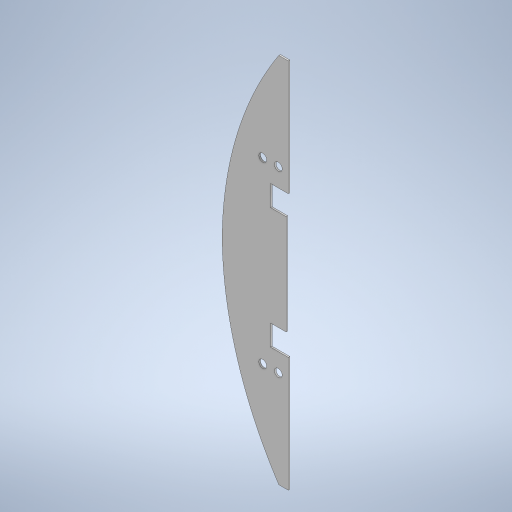
# Autodesk Inventor part: sensor2
Saved by Autodesk Inventor 2023 (Build 270158000, 158)
## iProperties
Created: 2023-08-10
Part Number: sensor2
Material: Genérico
Document SubType Name: Modeling
Designer: azeve
Density: 1 g/cm^3
Appearance: Padrão
Author: azeve
Autodesk Inventor part; units mm, degrees
ref_plane "YZ Plane" through (0, 0, 0) normal (1, 0, 0) x (0, 1, 0)
ref_plane "XZ Plane" through (0, 0, 0) normal (0, 1, 0) x (-1, 0, 0)
ref_plane "XY Plane" through (0, 0, 0) normal (0, 0, 1) x (1, 0, 0)
sketch "Esboço1" plane through (0, 0, 0) normal (0, 0, 1) x (1, 0, 0)
  line L0 (15.7389, -119.5954) -> (21.8039, -119.5954)
  line L1 (21.8039, -119.5954) -> (21.8039, -45.5852)
  line L2 (10.4016, -45.5852) -> (10.4016, -32.1476)
  line L3 (20.3752, -32.1476) -> (20.3752, 0.0017)
  arc A0 (-20.7435, 0.0017) -> (15.7389, -119.5954) centre (201.4548, 2.419) ccw
  circle A1 centre (15.3884, -57.4534) radius 2.5
  line L4 (21.8039, -45.5852) -> (10.4016, -45.5852)
  line L5 (20.3752, -32.1476) -> (10.4016, -32.1476)
  line L6 (20.3752, 0.0017) -> (13.075, 0.0017)
  arc A2 (15.7389, 119.5989) -> (-20.7435, 0.0017) centre (201.4548, -2.4155) ccw
  line L7 (20.3752, 32.1511) -> (20.3752, 0.0017)
  circle A3 centre (15.3884, 57.4569) radius 2.5
  line L8 (10.4016, 45.5887) -> (10.4016, 32.1511)
  line L9 (15.7389, 119.5989) -> (21.8039, 119.5989)
  line L10 (21.8039, 45.5887) -> (10.4016, 45.5887)
  line L11 (20.3752, 32.1511) -> (10.4016, 32.1511)
  line L12 (21.8039, 45.5887) -> (21.8039, 119.5989)
  circle A4 centre (5.3884, -57.4534) radius 2.5
  circle A5 centre (5.3884, 57.4569) radius 2.5
  point P0 (0, 0)
  dimension "d0" = 5
  dimension "d6" = 10
  dimension "d13" = 10
  constraints: 26 end point, 8 symmetric about line, 6 centre point, 5 horizontal, 4 point on circle, 1 parallel, 1 perpendicular, 1 vertical, 6 other
  measures "d0" diameter of A1
  measures "d6" distance of A1.centre A4.centre
  measures "d13" distance of A3.centre A5.centre
extrude "Extrusão1" add sketch "Esboço1" along normal blind 1
